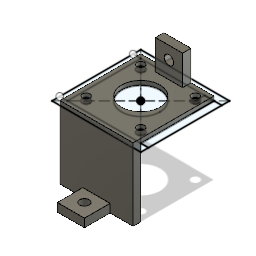
UppNiðurFesting v2 (Autodesk Fusion 360 design; units mm, degrees)
Autodesk Fusion 360 part; units mm, degrees
note: some values were not read from the file. Set by a fixed rule: which sketch regions a step uses.
sketch "Sketch1" plane through (0, 0, 0) normal (0, 1, 0) x (1, 0, 0)
  circle A0 centre (0, 0) radius 11.2
  line L0 (21.5, 21.5) -> (-21.5, 21.5)
  line L1 (-21.5, 21.5) -> (-21.5, -21.5)
  line L2 (-21.5, -21.5) -> (21.5, -21.5)
  line L3 (21.5, -21.5) -> (21.5, 21.5)
  line L4 (21.5, 21.5) -> (-21.5, -21.5) construction
  line L5 (-21.5, 21.5) -> (21.5, -21.5) construction
  line L6 (21.5, 21.5) -> (16, 21.5)
  line L7 (16, 21.5) -> (16, 16)
  circle A1 centre (16, 16) radius 2.2
  circle A2 centre (-16, 16) radius 2.2
  circle A3 centre (-16, -16) radius 2.2
  circle A4 centre (16, -16) radius 2.2
  line L8 (26, 26) -> (-26, 26)
  line L9 (-26, 26) -> (-26, -26)
  line L10 (-26, -26) -> (26, -26)
  line L11 (26, -26) -> (26, 26)
  line L12 (26, 26) -> (-26, -26) construction
  line L13 (-26, 26) -> (26, -26) construction
  line L14 (-21.5, -21.5) -> (-26, -21.5)
  line L15 (21.5, -21.5) -> (26, -21.5)
  line L16 (-21.5, 21.5) -> (-26, 21.5)
  line L17 (21.5, 21.5) -> (26, 21.5)
  dimension "d1" = 22.4
  dimension "d2" = 43
  dimension "d3" = 43
  dimension "d4" = 5.5
  dimension "d5" = 5.5
  dimension "d6" = 4.4
  dimension "d8" = 360
  dimension "d9" = 52
  dimension "d10" = 52
  constraint coincident A0.centre origin
  constraint horizontal L0
  constraint perpendicular L0 L1
  constraint parallel L0 L2
  constraint parallel L1 L3
  constraint coincident L4 A0.centre
  constraint coincident L5 A0.centre
  constraint perpendicular L3 L6
  constraint perpendicular L6 L7
  constraint coincident L7.end A1.centre
  constraint horizontal L8
  constraint perpendicular L8 L9
  constraint parallel L8 L10
  constraint parallel L9 L11
  constraint coincident L12 A0.centre
  constraint coincident L13 A0.centre
  constraint perpendicular L1 L14
  constraint coincident L11 L15.end
  constraint perpendicular L11 L15
  constraint perpendicular L1 L16
  constraint coincident L11 L17.end
  constraint perpendicular L11 L17
  measures "d1" diameter of A0
  measures "d2" distance of L1.end L2.end
  measures "d3" distance of L0.end L1.end
  measures "d4" distance of L0.start L6.end
  measures "d5" distance of L6.end L7.end
  measures "d6" diameter of A1
  measures "d9" distance of L9.end L10.end
  measures "d10" distance of L8.end L9.end
extrude "Extrude1" add sketch "Sketch1" along normal blind 5
extrude "Extrude7" add sketch "Sketch1" against normal blind 40 contours L2 L9 L10 L11 L14 L15
extrude "Extrude8" cut sketch "Sketch1" along normal blind 32 contours L0 L6 L8 L9 L11 L16 L17
sketch "Sketch7" plane through (0, 5, 0) normal (0, 1, 0) x (-1, 0, 0)
  line L0 (-26, -21.5) -> (26, -21.5)
  line L1 (26, -21.5) -> (26, 26)
  line L2 (26, 26) -> (-26, 26)
  line L3 (-26, 26) -> (-26, -21.5)
  circle A0 centre (16, 16) radius 2.2
  circle A1 centre (-16, 16) radius 2.2
  circle A2 centre (16, -16) radius 2.2
  circle A3 centre (0, 0) radius 11.2
  circle A4 centre (-16, -16) radius 2.2
  line L4 (0, -21.5) -> (8, -21.5)
  line L5 (8, -21.5) -> (-8, -21.5)
  line L6 (-8, -21.5) -> (-8, -16.5)
  line L7 (-8, -16.5) -> (8, -16.5)
  line L8 (8, -16.5) -> (8, -21.5)
  dimension "d48" = 8
  dimension "d49" = 16
  dimension "d50" = 5
  constraint midpoint L0 L4.start
  constraint parallel L0 L4
  constraint horizontal L5
  constraint vertical L6
  constraint horizontal L7
  constraint vertical L8
  measures "d48" distance of L4.start L4.end
  measures "d49" distance of L4.end L5.end
  measures "d50" distance of L4.end L7.end
extrude "Extrude9" add sketch "Sketch7" along normal blind 15 contours L0 L4 L5 L6 L7 L8
sketch "Sketch8" plane through (0, 0, -16.5) normal (0, 0, 1) x (1, 0, 0)
  line L0 (-8, 5) -> (8, 5)
  line L1 (8, 5) -> (8, 20)
  line L2 (8, 20) -> (-8, 20)
  line L3 (-8, 20) -> (-8, 5)
  line L4 (0, 20) -> (0, 12.5)
  circle A0 centre (0, 12.5) radius 2.75
  dimension "d53" = 5.5
  constraint midpoint L2 L4.start
  constraint perpendicular L2 L4
  constraint coincident L4.end A0.centre
  measures "d53" diameter of A0
extrude "Extrude10" cut sketch "Sketch8" against normal blind 14 contours A0
sketch "Sketch9" plane through (0, 0, 26) normal (0, 0, 1) x (1, 0, 0)
  line L0 (26, -40) -> (26, 5)
  line L1 (26, 5) -> (-26, 5)
  line L2 (-26, 5) -> (-26, -40)
  line L3 (-26, -40) -> (26, -40)
  line L4 (0, -40) -> (8, -40)
  line L5 (8, -40) -> (-8, -40)
  line L6 (-8, -40) -> (-8, -35)
  line L7 (-8, -35) -> (8, -35)
  line L8 (8, -35) -> (8, -40)
  dimension "d56" = 8
  dimension "d57" = 16
  dimension "d58" = 5
  constraint midpoint L3 L4.start
  constraint parallel L3 L4
  constraint horizontal L5
  constraint vertical L6
  constraint horizontal L7
  constraint vertical L8
  measures "d56" distance of L4.start L4.end
  measures "d57" distance of L4.end L5.end
  measures "d58" distance of L4.end L7.end
extrude "Extrude11" add sketch "Sketch9" along normal blind 15 contours L3 L4 L5 L6 L7 L8
sketch "Sketch10" plane through (0, -35, 0) normal (0, 1, 0) x (-1, 0, 0)
  line L0 (-8, 26) -> (8, 26)
  line L1 (8, 26) -> (8, 41)
  line L2 (8, 41) -> (-8, 41)
  line L3 (-8, 41) -> (-8, 26)
  line L4 (0, 41) -> (0, 33)
  circle A0 centre (0, 33) radius 2.75
  dimension "d61" = 5.5
  constraint midpoint L2 L4.start
  constraint perpendicular L2 L4
  constraint coincident L4.end A0.centre
  measures "d61" diameter of A0
extrude "Extrude12" cut sketch "Sketch10" against normal blind 11 contours A0
extrude "Extrude13" cut sketch "Sketch1" along normal blind 6 contours L3 L11 L15 L17 | L1 L9 L14 L16
sketch "Sketch11" plane through (0, 0, 21.5) normal (0, 0, -1) x (-1, 0, 0)
  line L0 (-26, 5) -> (-26, -40)
  line L1 (-26, -40) -> (26, -40)
  line L2 (26, -40) -> (26, 5)
  line L3 (26, 5) -> (21.5, 5)
  line L4 (21.5, 5) -> (21.5, 0)
  line L5 (21.5, 0) -> (-21.5, 0)
  line L6 (-21.5, 0) -> (-21.5, 5)
  line L7 (-21.5, 5) -> (-26, 5)
  line L8 (21.5, 0) -> (21.5, -40)
  line L9 (-21.5, 0) -> (-21.5, -40)
  constraint coincident L4.end L5.start
  constraint coincident L1 L8.end
  constraint perpendicular L1 L8
  constraint coincident L5.end L6.start
  constraint coincident L1 L9.end
  constraint perpendicular L1 L9
extrude "Extrude14" cut sketch "Sketch11" against normal blind 15 contours L0 L1 L6 L7 L9 | L1 L2 L3 L4 L8
extrude "Extrude15" cut 1 faces at (4.8761, 5, 23.24) along direction (0, -1, 0) blind 2.5
